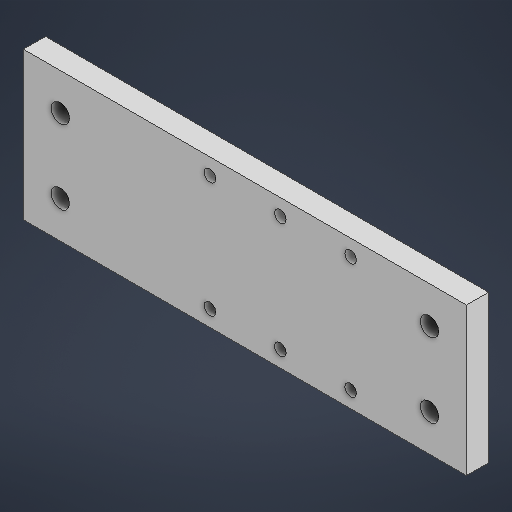
# Autodesk Inventor part: motor_bracket_base2
Saved by Autodesk Inventor 2026 (Build 300175050, 175E)
## iProperties
Created: 2025-11-11
Part Number: motor_bracket_base2
Material: Generic
Document SubType Name: Modeling
Designer: habbo
Density: 1 g/cm^3
Appearance: Default
Author: habbo
Autodesk Inventor part; units mm, degrees
ref_plane "YZ Plane" through (0, 0, 0) normal (1, 0, 0) x (0, 1, 0)
ref_plane "XZ Plane" through (0, 0, 0) normal (0, 1, 0) x (-1, 0, 0)
ref_plane "XY Plane" through (0, 0, 0) normal (0, 0, 1) x (1, 0, 0)
sketch "Sketch1" plane through (0, 0, 0) normal (0, 0, 1) x (1, 0, 0)
  line L0 (-60, -20) -> (60, -20)
  line L1 (60, -20) -> (60, 20)
  line L2 (60, 20) -> (-60, 20)
  line L3 (-60, 20) -> (-60, -20)
  line L4 (-60, -20) -> (60, 20) construction
  line L5 (60, -20) -> (-60, 20) construction
  circle A0 centre (28.637, -15.621) radius 1.5875
  circle A1 centre (9.587, -15.621) radius 1.5875
  circle A2 centre (-9.463, -15.621) radius 1.5875
  circle A3 centre (28.637, 15.621) radius 1.5875
  circle A4 centre (9.587, 15.621) radius 1.5875
  circle A5 centre (-9.463, 15.621) radius 1.5875
  circle A6 centre (50, -10) radius 2.5
  circle A7 centre (50, 10) radius 2.5
  circle A8 centre (-50, -10) radius 2.5
  circle A9 centre (-50, 10) radius 2.5
  point P0 (0, 0)
  dimension "d0" = 120
  dimension "d1" = 40
  dimension "d4" = 3.175
  dimension "d5" = 3.175
  dimension "d6" = 3.175
  dimension "d7" = 3.175
  dimension "d8" = 3.175
  dimension "d9" = 3.175
  dimension "d10" = 31.242
  dimension "d11" = 19.05
  dimension "d12" = 19.05
  dimension "d13" = 31.363
  dimension "d14" = 5
  dimension "d15" = 5
  dimension "d16" = 5
  dimension "d17" = 5
  dimension "d20" = 10
  dimension "d21" = 10
  dimension "d22" = 20
  dimension "d23" = 10
  dimension "d26" = 4.379
  constraints: 12 end point, 10 centre point, 6 horizontal alignment, 5 vertical alignment, 2 midpoint, 2 parallel, 1 horizontal, 1 perpendicular
  measures "d0" distance of L2.end L1.end
  measures "d1" distance of L1.end L0.end
  measures "d4" diameter of A0
  measures "d5" diameter of A1
  measures "d6" diameter of A2
  measures "d7" diameter of A3
  measures "d8" diameter of A4
  measures "d9" diameter of A5
  measures "d10" distance of A3.centre A0.centre
  measures "d11" distance of A1.centre A0.centre
  measures "d12" distance of A2.centre A1.centre
  measures "d13" distance from line of L1 A0.centre
  measures "d14" diameter of A6
  measures "d15" diameter of A7
  measures "d16" diameter of A8
  measures "d17" diameter of A9
  measures "d20" distance from line of L1 A6.centre
  measures "d21" distance from line of A8.centre L3
  measures "d22" distance of A7.centre A6.centre
  measures "d23" distance from line of L2 A7.centre
  measures "d26" distance from line of L0 A0.centre
extrude "Extrusion2" add sketch "Sketch1" along normal mid plane 6
body "Solid2"
